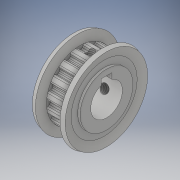
# Autodesk Inventor part: MTP16XL025-A-N12_b
Saved by Autodesk Inventor 2019 (Build 230136000, 136)
## iProperties
Created: 2023-12-31
Part Number: MTP16XL025-A-N12_b
Material: Generic
Catalog Web Link: www.cadenas.de
Description: ATP__XL025, ATP__XL031, ATP__ XL037, ATP__XL050, BTP__XL025, BTP__XL031, BTP__XL037, BTP__XL050, KTP__XL025, KTP__XL031, KTP__ XL037, KTP__XL050, NTP__XL025, NTP__XL031, NTP__ XL037, NTP__XL050, MTP__XL025, MTP__ XL037, MTP__XL050, MTPB__XL025, MTPB__ XL037, MTPB__XL050, MTPP__XL025, MTPP__ XL037, MTPP__XL050, STP__XL025, STP__XL031, STP__ XL037, STP__XL050, KATP__XL025, KATP__XL031, KATP__ XL037, KATP__XL050, KKTP__XL025, KKTP__XL031, KKTP__ XL037, KKTP__XL050_body-Timing Pulleys XL Type
Vendor: MISUMI
Document SubType Name: Modeling
Designer: psAdmin
Manufacturer: MISUMI
Mass: 4.98288 g
Surface Area: 37.8278 cm^2
Volume: 4.98288 cm^3
Density: 1 g/cm^3
Appearance: PSOLRGB-175-175-175
Category: PARTsolutions
Company: MISUMI
Title: MTP16XL025-A-N12
Author: Cadenas PARTsolutions
Comments: Timing Pulleys XL Type
PSOL_IDENT_0: {$CADENAS_DATA/23d-libs/misumi/metric/51_timing_pulleys/mtp_xl/mtp_xl.prj},887 {VTYP=3D},{NB=MTP16XL
PSOL_IDENT_1: 025-A-N12_b},{LINA=MTP16XL025-A-N12},{NN=ATP__XL025, ATP__XL031, ATP__ XL037, ATP__XL050, BTP__XL025
PSOL_IDENT_2: , BTP__XL031, BTP__XL037, BTP__XL050, KTP__XL025, KTP__XL031, KTP__ XL037, KTP__XL050, NTP__XL025, N
PSOL_IDENT_3: TP__XL031, NTP__ XL037, NTP__XL050, MTP__XL025, MTP__ XL037, MTP__XL050, MTPB__XL025, MTPB__ XL037,
PSOL_IDENT_4: MTPB__XL050, MTPP__XL025, MTPP__ XL037, MTPP__XL050, STP__XL025, STP__XL031, STP__ XL037, STP__XL050
PSOL_IDENT_5: , KATP__XL025, KATP__XL031, KATP__ XL037, KATP__XL050, KKTP__XL025, KKTP__XL031, KKTP__ XL037, KKTP_
PSOL_IDENT_6: _XL050_body},{DATE=06.01.2023 09:07:12},{GEOMDATE=06.01.2023 09:06:51},{VERSION=},{LINEID=30},{WBVAR=
PSOL_IDENT_7: MATP,ST,TNW,PS,SBS,DD,Z,J,Q,R,S,T,ALT1,ALT2,M,QSC,QFC,QTC,ALT3,K,KSC,KFC,KTC,ALT4,ZM,ZSC,ZFC,ZTC,ALT
PSOL_IDENT_8: 5,ALT6,ALT7,FC,ALT8,SRG,ALT9,BTC,TL,ALT10,TPC,ALT11,BC,ALT12,SLH,ALT13,BN},{WBNUMERIC=DD,Z,J,Q,R,S,T
PSOL_IDENT_9: ,QSC,QFC,QTC,K,KSC,KFC,KTC,ZSC,ZFC,ZTC,FC,SRG,BTC,TL,BC,SLH,BN}  {NB=MTP16XL025-A-N12_b},{LINA=MTP16
PSOL_IDENT_10: XL025-A-N12},{KT=DUMMY},{PN=MTP16XL025-A-N12},{TYPE=MTP},{MATP=S45C},{MATPALG= 'A2017','Aluminum All
PSOL_IDENT_11: oy 2000 series','S45C','1045 Carbon Steel Equivalent','SUS304','SUS304', 'A6000', '6000 Series Alumi
PSOL_IDENT_12: num Alloy' },{ST=-},{STALG= '-','-','BO','Black Oxide','ENP','Electroless Nickel Plating' },{NT=16},
PSOL_IDENT_13: {TNW=XL025},{TNWALG= 'XL025','XL031','XL037','XL050' },{BW=6.4mm (1/4inch)},{PS=A},{PSALG= 'A','B' }
PSOL_IDENT_14: ,{SBS=N},{SBSALG= 'H','Round Hole','P','Round Hole + Tap','N','New JIS Keywayed Bore + Tap (Standard
PSOL_IDENT_15: )','NK','New JIS Keywayed Bore + Tap (width 4.0mm, height 1.8mm)','C','Old JIS Keywayed Bore + Tap','
PSOL_IDENT_16: V','Stepped Hole','Y','Both Ends Stepped Hole','WB','Double Stepped Hole' },{DD=12.00},{DDALG=[8:8/1
PSOL_IDENT_17: ],[10:13/1]},{DDHA=[5:6/1],6.35,[7:12/1],12.7,[13:16/1]},{DDPA=[5:6/1],6.35,[7:12/1],12.7,[13:13/1]}
PSOL_IDENT_18: ,{DDNA=[8:8/1],[10:13/1]},{DDNK=[10:10/1]},{DDCA=[10,12]},{DDVA=[5:6/1],6.35,[7:12/1],12.7,[13:14/1]
PSOL_IDENT_19: },{DDY=[5:14/1]},{DDWB=[5:12/1]},{DDHB=},{DDPB=},{DDNB=},{DDCB=},{DDVFB=},{Z=0},{ZALG=[0]},{ZMIN=14.
PSOL_IDENT_20: 000},{ZAMAX=16.000},{ZBMAX=0.000},{DDZ=12.000},{J=0.0},{JALG=[0]},{JMIN=2.000},{JMAX=10.5},{JPN=},{Q=
PSOL_IDENT_21: 0},{QALG=[0]},{QRMIN=14.000},{QRMAX=16},{WBQMIN=16.000},{R=0},{RALG=[0]},{WBRMAX=-2.000},{S=0.0},{SA
PSOL_IDENT_22: LG=[0]},{SMAX=6.5},{T=0.0},{TALG=[0]},{TMAX=8},{SBSPN=-N12},{A=7.5},{W=12.5},{L=0},{PD=25.87},{OD=25
PSOL_IDENT_23: .36},{D=0},{DALG=17.000},{DE=20},{F=32},{E=20},{TT=1.6},{BBK=4.000},{TTK=1.8},{ALT1=},{ANG=112.500},
PSOL_IDENT_24: {ALT1ALG= '','w/o KC90 (Set Screw Angle)','KC90','with KC90 (Set Screw Angle)' },{ALT1PN=},{ALT2=},{
PSOL_IDENT_25: ALT2ALG= '','Not applicable' },{M=N/A},{MALG= 'N/A' },{MFTALG= 'N/A' },{MSALG= 'N/A' },{M3D=0.000},{
PSOL_IDENT_26: KDML=0.000},{ML=0.000},{MUL=0.000},{PITCH=0.000},{QSC=0.0},{QSCALG=0},{QFC=0.0},{QFCALG=0},{QTC=0.0}
PSOL_IDENT_27: ,{QTCALG=0},{QPCDMIN=0.000},{QPCDMINALG=0.000},{QPCDMAX=16.000},{ALT2PN=},{TAP=0.000},{ALT3=},{ALT3A
PSOL_IDENT_28: LG= '','Not applicable' },{K=0.0},{KALG=0},{KMIN=4.000},{KFTMAX=0.000},{KSMAX=0.000},{KSC=0.0},{KSCA
PSOL_IDENT_29: LG=0},{KFC=0.0},{KFCALG=0},{KTC=0.0},{KTCALG=0},{KSCMIN=16.000},{KPCDMIN=16.000},{KPCDMAX=16.000},{A
PSOL_IDENT_30: LT3PN=},{ALT4=},{ALT4ALG= '','Not applicable' },{ALT4MIN=22.500},{ALT4MAX=9.500},{ZM=N/A},{ZMALG= 'N
PSOL_IDENT_31: /A' },{ZMFTALG= 'N/A' },{ZMSALG= 'N/A' },{ZMDD1=0.0},{ZMDD2=0.0},{ZMHH=0.0},{ZSC=0.0},{ZSCALG=[0]},{
PSOL_IDENT_32: ZFC=0.0},{ZFCALG=[0]},{ZTC=0.0},{ZTCALG=[0]},{ZPCDMIN=0.000},{ZPCDMINALG=0.000},{ZPCDMAX=16.000},{AL
PSOL_IDENT_33: T4PN=},{ALT5=},{ALT5ALG= '','w/o Flange not Attached','NFC','with NFC (Flange not Attached)' },{ALT5
PSOL_IDENT_34: PN=},{ALT6=},{ALT6ALG= '','w/o Flange Attached on One Side Only','RFC','with RFC (Flange Attached on
PSOL_IDENT_35: The Boss Side Only)','LFC','with LFC (Flange Attached on The Opposite Side Only)' },{ALT6PN=},{ALT7=
PSOL_IDENT_36: },{ALT7ALG= '','w/o FC (Flange Cut)','FC','with FC (Flange Cut)' },{FC=0.0},{FCALG=0},{FCMIN=26.5},{
PSOL_IDENT_37: FCMAX=30.0},{ALT7PN=},{ALT8=},{ALT8ALG= '','Not applicable' },{ALT8ALGALG=16.000},{ALT8DD2=0.000},{A
PSOL_IDENT_38: LT8MM=0.000},{ALT8NN=0.000},{QC=0.000},{KC=0.000},{ZC=0.000},{SRG=0.0},{SRGALG=[0]},{SRGMAX=0.000},{
PSOL_IDENT_39: DD2=0.0},{MM=0.00},{NN=0.00},{ALT8PN=},{ALT9=},{ALT9ALG= '','Not applicable' },{BTC9=14.000},{TL9=1.
PSOL_IDENT_40: 000},{BTC=0},{BTCALG=[0]},{TL=0.0},{TLALG=0},{TLMIN=1.000},{TLMAX=-13.000},{BTCL=0},{BTCD=0},{ALT9PN=
PSOL_IDENT_41: },{WLBCTL=12.500},{ALT10=},{ALT10ALG= '','w/o TPC (Tapped Hole Dimension)','TPC','with TPC (Tapped H
PSOL_IDENT_42: ole Dimension)' },{TPC=N/A},{TPCALG= 'N/A' },{TPCM=4.000},{ALT10PN=},{ALT11=},{ALT11ALG= '','Not app
PSOL_IDENT_43: licable' },{BC=0.0},{BCALG=0},{BCMIN=7},{BCMAX=-13},{M1WBC=6.25},{ALT11PN=},{KTT=4.88},{ALT12=},{ALT
PSOL_IDENT_44: 12ALG= '','w/o SLH (Set Screw Length)','SLH','with SLH (Set Screw Length)' },{SLHALG=[0]},{SLH=0},{A
PSOL_IDENT_45: LT12PN=},{ALT13=},{ALT13ALG= '', 'Not applicable' },{BN=0.0},{BNALG=0},{BNMIN=-12},{BNMAX=-2.5},{ALT
PSOL_IDENT_46: 13PN=},{AC=M4x3},{M1=4.000},{M1L=3.000},{KEYA=1.000},{KEYB=0.000},{KEYM=1.000}
NB: MTP16XL025-A-N12_b
NN: 0
NT: 16
NBSYN: $PN._b
LINA: MTP16XL025-A-N12
CATALOG: Misumi
PN: MTP16XL025-A-N12
MATP: 1045 Carbon Steel Equivalent
ST: -
TNW: XL025
BW: 6.4mm (1/4inch)
PS: A
SBS: New JIS Keywayed Bore + Tap (Standard)
DD: 12
Z: 0
J: 0
Q: 0
R: 0
S: 0
T: 0
A: 7.5
W: 12.5
L: 0
PD: 25.87
OD: 25.36
D: 0
F: 32
E: 20
TT: 1.6
ALT1: w/o KC90 (Set Screw Angle)
ALT2: Not applicable
M: N/A
QSC: 0
QFC: 0
QTC: 0
ALT3: Not applicable
K: 0
KSC: 0
KFC: 0
KTC: 0
ALT4: Not applicable
ZM: N/A
ZMDD1: 0
ZMDD2: 0
ZMHH: 0
ZSC: 0
ZFC: 0
ZTC: 0
ALT5: w/o Flange not Attached
ALT6: w/o Flange Attached on One Side Only
ALT7: w/o FC (Flange Cut)
FC: 0
ALT8: Not applicable
SRG: 0
DD2: 0
MM: 0
ALT9: Not applicable
BTC: 0
TL: 0
BTCL: 0
BTCD: 0
ALT10: w/o TPC (Tapped Hole Dimension)
TPC: N/A
ALT11: Not applicable
BC: 0
ALT12: w/o SLH (Set Screw Length)
SLH: 0
ALT13: Not applicable
BN: 0
AC: M4x3
SUPPLIER: MISUMI
ARTICLENO: MTP16XL025-A-N12_b
BOMINFO: MTP16XL025-A-N12
CREATOR: CADENAS GmbH
Autodesk Inventor part; units mm, degrees
sketch "_____2" plane through (0, 0, 0) normal (0, 0, 1) x (1, 0, 0)
  line L0 (12.5, 0) -> (0, 0)
  line L1 (0, 0) -> (0, 10)
  line L2 (0, 10) -> (0.9, 10)
  line L3 (0.9, 10) -> (0.9, 12.469356)
  line L4 (0.9, 12.469356) -> (0.064927, 15.58589)
  line L5 (0.064927, 15.58589) -> (1.610409, 16)
  line L6 (1.610409, 16) -> (2.5, 12.68)
  line L7 (2.5, 12.68) -> (10, 12.68)
  line L8 (10, 12.68) -> (10.889591, 16)
  line L9 (10.889591, 16) -> (12.435073, 15.58589)
  line L10 (12.435073, 15.58589) -> (11.6, 12.469356)
  line L11 (11.6, 12.469356) -> (11.6, 10)
  line L12 (11.6, 10) -> (12.5, 10)
  line L13 (12.5, 10) -> (12.5, 0)
  line L14 (12.5, 0) -> (0, 0)
  constraints: 30 end point
revolve "Revolution1" add sketch "_____2" angle 360 about axis through (12.5, 0, 0) along (1, 0, 0)
sketch "Sketch2" plane through (12.5, 0, 0) normal (1, 0, 0) x (0, 0, -1)
  point P0 (0, 0)
hole "Hole1" at (12.5, 0, 0) direction (-1, 0, 0) diameter 12 depth 12.5
sketch "_____6" plane through (2.5, 0, 0) normal (1, 0, 0) x (0, 0, -1)
  arc A0 (-12.686458, 2.523493) -> (-12.686458, -2.523493) centre (0, 0) ccw
  arc A1 (-12.686458, -2.523493) -> (-10.755059, -7.186301) centre (0, 0) ccw
  arc A2 (-10.755059, -7.186301) -> (-7.186301, -10.755059) centre (0, 0) ccw
  arc A3 (-7.186301, -10.755059) -> (-2.523493, -12.686458) centre (0, 0) ccw
  arc A4 (-2.523493, -12.686458) -> (2.523493, -12.686458) centre (0, 0) ccw
  arc A5 (2.523493, -12.686458) -> (7.186301, -10.755059) centre (0, 0) ccw
  arc A6 (7.186301, -10.755059) -> (10.755059, -7.186301) centre (0, 0) ccw
  arc A7 (10.755059, -7.186301) -> (12.686458, -2.523493) centre (0, 0) ccw
  arc A8 (12.686458, -2.523493) -> (12.686458, 2.523493) centre (0, 0) ccw
  arc A9 (12.686458, 2.523493) -> (10.755059, 7.186301) centre (0, 0) ccw
  arc A10 (10.755059, 7.186301) -> (7.186301, 10.755059) centre (0, 0) ccw
  arc A11 (7.186301, 10.755059) -> (2.523493, 12.686458) centre (0, 0) ccw
  arc A12 (2.523493, 12.686458) -> (-2.523493, 12.686458) centre (0, 0) ccw
  arc A13 (-2.523493, 12.686458) -> (-7.186301, 10.755059) centre (0, 0) ccw
  arc A14 (-7.186301, 10.755059) -> (-10.755059, 7.186301) centre (0, 0) ccw
  arc A15 (-10.755059, 7.186301) -> (-12.686458, 2.523493) centre (0, 0) ccw
  arc A16 (-12.216815, -1.080185) -> (-12.563409, -1.715564) centre (-11.959018, -1.633033) ccw
  arc A17 (-12.563409, -1.715564) -> (-12.436357, -2.473745) centre (0, 0) ccw
  arc A18 (-12.436357, -2.473745) -> (-12.263594, -3.222834) centre (0, 0) ccw
  arc A19 (-12.263594, -3.222834) -> (-11.700234, -3.677212) centre (-11.673626, -3.067792) ccw
  line L0 (-11.700234, -3.677212) -> (-11.052822, -3.705478)
  arc A20 (-10.511015, -4.093528) -> (-11.052822, -3.705478) centre (-11.079429, -4.314898) ccw
  arc A21 (-10.511015, -4.093528) -> (-10.326971, -4.537849) centre (0, 0) ccw
  arc A22 (-10.435694, -5.195356) -> (-10.326971, -4.537849) centre (-10.885433, -4.783246) ccw
  line L1 (-10.435694, -5.195356) -> (-10.873496, -5.673133)
  arc A23 (-10.873496, -5.673133) -> (-10.950558, -6.392783) centre (-10.423757, -6.085244) ccw
  arc A24 (-10.950558, -6.392783) -> (-10.543035, -7.044631) centre (0, 0) ccw
  arc A25 (-10.543035, -7.044631) -> (-10.096758, -7.670585) centre (0, 0) ccw
  arc A26 (-10.096758, -7.670585) -> (-9.402399, -7.874786) centre (-9.611031, -7.301574) ccw
  line L2 (-9.402399, -7.874786) -> (-8.79345, -7.653147)
  arc A27 (-8.144386, -7.804318) -> (-8.79345, -7.653147) centre (-8.584818, -8.22636) ccw
  arc A28 (-8.144386, -7.804318) -> (-7.804318, -8.144386) centre (0, 0) ccw
  arc A29 (-7.653147, -8.79345) -> (-7.804318, -8.144386) centre (-8.22636, -8.584818) ccw
  line L3 (-7.653147, -8.79345) -> (-7.874786, -9.402399)
  arc A30 (-7.874786, -9.402399) -> (-7.670585, -10.096758) centre (-7.301574, -9.611031) ccw
  arc A31 (-7.670585, -10.096758) -> (-7.044631, -10.543035) centre (0, 0) ccw
  arc A32 (-7.044631, -10.543035) -> (-6.392783, -10.950558) centre (0, 0) ccw
  arc A33 (-6.392783, -10.950558) -> (-5.673133, -10.873496) centre (-6.085244, -10.423757) ccw
  line L4 (-5.673133, -10.873496) -> (-5.195356, -10.435694)
  arc A34 (-4.537848, -10.326971) -> (-5.195356, -10.435694) centre (-4.783246, -10.885433) ccw
  arc A35 (-4.537848, -10.326971) -> (-4.093528, -10.511015) centre (0, 0) ccw
  arc A36 (-3.705478, -11.052822) -> (-4.093528, -10.511015) centre (-4.314898, -11.079429) ccw
  line L5 (-3.705478, -11.052822) -> (-3.677212, -11.700234)
  arc A37 (-3.677212, -11.700234) -> (-3.222834, -12.263594) centre (-3.067792, -11.673626) ccw
  arc A38 (-3.222834, -12.263594) -> (-2.473745, -12.436357) centre (0, 0) ccw
  arc A39 (-2.473745, -12.436357) -> (-1.715564, -12.563409) centre (0, 0) ccw
  arc A40 (-1.715564, -12.563409) -> (-1.080185, -12.216815) centre (-1.633033, -11.959018) ccw
  line L6 (-1.080185, -12.216815) -> (-0.806316, -11.629501)
  arc A41 (-0.240464, -11.277437) -> (-0.806316, -11.629501) centre (-0.253468, -11.887298) ccw
  arc A42 (-0.240464, -11.277437) -> (0.240464, -11.277437) centre (0, 0) ccw
  arc A43 (0.806316, -11.629501) -> (0.240464, -11.277437) centre (0.253468, -11.887298) ccw
  line L7 (0.806316, -11.629501) -> (1.080185, -12.216815)
  arc A44 (1.080185, -12.216815) -> (1.715564, -12.563409) centre (1.633033, -11.959018) ccw
  arc A45 (1.715564, -12.563409) -> (2.473745, -12.436357) centre (0, 0) ccw
  arc A46 (2.473745, -12.436357) -> (3.222834, -12.263594) centre (0, 0) ccw
  arc A47 (3.222834, -12.263594) -> (3.677212, -11.700234) centre (3.067792, -11.673626) ccw
  line L8 (3.677212, -11.700234) -> (3.705478, -11.052822)
  arc A48 (4.093528, -10.511015) -> (3.705478, -11.052822) centre (4.314898, -11.079429) ccw
  arc A49 (4.093528, -10.511015) -> (4.537849, -10.326971) centre (0, 0) ccw
  arc A50 (5.195356, -10.435694) -> (4.537849, -10.326971) centre (4.783246, -10.885433) ccw
  line L9 (5.195356, -10.435694) -> (5.673133, -10.873496)
  arc A51 (5.673133, -10.873496) -> (6.392783, -10.950558) centre (6.085244, -10.423757) ccw
  arc A52 (6.392783, -10.950558) -> (7.044631, -10.543035) centre (0, 0) ccw
  arc A53 (7.044631, -10.543035) -> (7.670585, -10.096758) centre (0, 0) ccw
  arc A54 (7.670585, -10.096758) -> (7.874786, -9.402399) centre (7.301574, -9.611031) ccw
  line L10 (7.874786, -9.402399) -> (7.653147, -8.79345)
  arc A55 (7.804318, -8.144386) -> (7.653147, -8.79345) centre (8.22636, -8.584818) ccw
  arc A56 (7.804318, -8.144386) -> (8.144386, -7.804318) centre (0, 0) ccw
  arc A57 (8.79345, -7.653147) -> (8.144386, -7.804318) centre (8.584818, -8.22636) ccw
  line L11 (8.79345, -7.653147) -> (9.402399, -7.874786)
  arc A58 (9.402399, -7.874786) -> (10.096758, -7.670585) centre (9.611031, -7.301574) ccw
  arc A59 (10.096758, -7.670585) -> (10.543035, -7.044631) centre (0, 0) ccw
  arc A60 (10.543035, -7.044631) -> (10.950558, -6.392783) centre (0, 0) ccw
  arc A61 (10.950558, -6.392783) -> (10.873496, -5.673133) centre (10.423757, -6.085244) ccw
  line L12 (10.873496, -5.673133) -> (10.435694, -5.195356)
  arc A62 (10.326971, -4.537848) -> (10.435694, -5.195356) centre (10.885433, -4.783246) ccw
  arc A63 (10.326971, -4.537848) -> (10.511015, -4.093528) centre (0, 0) ccw
  arc A64 (11.052822, -3.705478) -> (10.511015, -4.093528) centre (11.079429, -4.314898) ccw
  line L13 (11.052822, -3.705478) -> (11.700234, -3.677212)
  arc A65 (11.700234, -3.677212) -> (12.263594, -3.222834) centre (11.673626, -3.067792) ccw
  arc A66 (12.263594, -3.222834) -> (12.436357, -2.473745) centre (0, 0) ccw
  arc A67 (12.436357, -2.473745) -> (12.563409, -1.715564) centre (0, 0) ccw
  arc A68 (12.563409, -1.715564) -> (12.216815, -1.080185) centre (11.959018, -1.633033) ccw
  line L14 (12.216815, -1.080185) -> (11.629501, -0.806316)
  arc A69 (11.277437, -0.240464) -> (11.629501, -0.806316) centre (11.887298, -0.253468) ccw
  arc A70 (11.277437, -0.240464) -> (11.277437, 0.240464) centre (0, 0) ccw
  arc A71 (11.629501, 0.806316) -> (11.277437, 0.240464) centre (11.887298, 0.253468) ccw
  line L15 (11.629501, 0.806316) -> (12.216815, 1.080185)
  arc A72 (12.216815, 1.080185) -> (12.563409, 1.715564) centre (11.959018, 1.633033) ccw
  arc A73 (12.563409, 1.715564) -> (12.436357, 2.473745) centre (0, 0) ccw
  arc A74 (12.436357, 2.473745) -> (12.263594, 3.222834) centre (0, 0) ccw
  arc A75 (12.263594, 3.222834) -> (11.700234, 3.677212) centre (11.673626, 3.067792) ccw
  line L16 (11.700234, 3.677212) -> (11.052822, 3.705478)
  arc A76 (10.511015, 4.093528) -> (11.052822, 3.705478) centre (11.079429, 4.314898) ccw
  arc A77 (10.511015, 4.093528) -> (10.326971, 4.537848) centre (0, 0) ccw
  arc A78 (10.435694, 5.195356) -> (10.326971, 4.537848) centre (10.885433, 4.783246) ccw
  line L17 (10.435694, 5.195356) -> (10.873496, 5.673133)
  arc A79 (10.873496, 5.673133) -> (10.950558, 6.392783) centre (10.423757, 6.085244) ccw
  arc A80 (10.950558, 6.392783) -> (10.543035, 7.044631) centre (0, 0) ccw
  arc A81 (10.543035, 7.044631) -> (10.096758, 7.670585) centre (0, 0) ccw
  arc A82 (10.096758, 7.670585) -> (9.402399, 7.874786) centre (9.611031, 7.301574) ccw
  line L18 (9.402399, 7.874786) -> (8.79345, 7.653147)
  arc A83 (8.144386, 7.804318) -> (8.79345, 7.653147) centre (8.584818, 8.22636) ccw
  arc A84 (8.144386, 7.804318) -> (7.804318, 8.144386) centre (0, 0) ccw
  arc A85 (7.653147, 8.79345) -> (7.804318, 8.144386) centre (8.22636, 8.584818) ccw
  line L19 (7.653147, 8.79345) -> (7.874786, 9.402399)
  arc A86 (7.874786, 9.402399) -> (7.670585, 10.096758) centre (7.301574, 9.611031) ccw
  arc A87 (7.670585, 10.096758) -> (7.044631, 10.543035) centre (0, 0) ccw
  arc A88 (7.044631, 10.543035) -> (6.392783, 10.950558) centre (0, 0) ccw
  arc A89 (6.392783, 10.950558) -> (5.673133, 10.873496) centre (6.085244, 10.423757) ccw
  line L20 (5.673133, 10.873496) -> (5.195356, 10.435694)
  arc A90 (4.537848, 10.326971) -> (5.195356, 10.435694) centre (4.783246, 10.885433) ccw
  arc A91 (4.537848, 10.326971) -> (4.093528, 10.511015) centre (0, 0) ccw
  arc A92 (3.705478, 11.052822) -> (4.093528, 10.511015) centre (4.314898, 11.079429) ccw
  line L21 (3.705478, 11.052822) -> (3.677212, 11.700234)
  arc A93 (3.677212, 11.700234) -> (3.222834, 12.263594) centre (3.067792, 11.673626) ccw
  arc A94 (3.222834, 12.263594) -> (2.473745, 12.436357) centre (0, 0) ccw
  arc A95 (2.473745, 12.436357) -> (1.715564, 12.563409) centre (0, 0) ccw
  arc A96 (1.715564, 12.563409) -> (1.080185, 12.216815) centre (1.633033, 11.959018) ccw
  line L22 (1.080185, 12.216815) -> (0.806316, 11.629501)
  arc A97 (0.240465, 11.277437) -> (0.806316, 11.629501) centre (0.253468, 11.887298) ccw
  arc A98 (0.240465, 11.277437) -> (-0.240465, 11.277437) centre (0, 0) ccw
  arc A99 (-0.806316, 11.629501) -> (-0.240465, 11.277437) centre (-0.253468, 11.887298) ccw
  line L23 (-0.806316, 11.629501) -> (-1.080185, 12.216815)
  arc A100 (-1.080185, 12.216815) -> (-1.715564, 12.563409) centre (-1.633033, 11.959018) ccw
  arc A101 (-1.715564, 12.563409) -> (-2.473745, 12.436357) centre (0, 0) ccw
  arc A102 (-2.473745, 12.436357) -> (-3.222834, 12.263594) centre (0, 0) ccw
  arc A103 (-3.222834, 12.263594) -> (-3.677212, 11.700234) centre (-3.067792, 11.673626) ccw
  line L24 (-3.677212, 11.700234) -> (-3.705478, 11.052822)
  arc A104 (-4.093528, 10.511015) -> (-3.705478, 11.052822) centre (-4.314898, 11.079429) ccw
  arc A105 (-4.093528, 10.511015) -> (-4.537849, 10.326971) centre (0, 0) ccw
  arc A106 (-5.195356, 10.435694) -> (-4.537849, 10.326971) centre (-4.783246, 10.885433) ccw
  line L25 (-5.195356, 10.435694) -> (-5.673133, 10.873496)
  arc A107 (-5.673133, 10.873496) -> (-6.392783, 10.950558) centre (-6.085244, 10.423757) ccw
  arc A108 (-6.392783, 10.950558) -> (-7.044631, 10.543035) centre (0, 0) ccw
  arc A109 (-7.044631, 10.543035) -> (-7.670585, 10.096758) centre (0, 0) ccw
  arc A110 (-7.670585, 10.096758) -> (-7.874786, 9.402399) centre (-7.301574, 9.611031) ccw
  line L26 (-7.874786, 9.402399) -> (-7.653147, 8.79345)
  arc A111 (-7.804318, 8.144386) -> (-7.653147, 8.79345) centre (-8.22636, 8.584818) ccw
  arc A112 (-7.804318, 8.144386) -> (-8.144386, 7.804318) centre (0, 0) ccw
  arc A113 (-8.79345, 7.653147) -> (-8.144386, 7.804318) centre (-8.584818, 8.22636) ccw
  line L27 (-8.79345, 7.653147) -> (-9.402399, 7.874786)
  arc A114 (-9.402399, 7.874786) -> (-10.096758, 7.670585) centre (-9.611031, 7.301574) ccw
  arc A115 (-10.096758, 7.670585) -> (-10.543035, 7.044631) centre (0, 0) ccw
  arc A116 (-10.543035, 7.044631) -> (-10.950558, 6.392783) centre (0, 0) ccw
  arc A117 (-10.950558, 6.392783) -> (-10.873496, 5.673133) centre (-10.423757, 6.085244) ccw
  line L28 (-10.873496, 5.673133) -> (-10.435694, 5.195356)
  arc A118 (-10.326971, 4.537848) -> (-10.435694, 5.195356) centre (-10.885433, 4.783246) ccw
  arc A119 (-10.326971, 4.537848) -> (-10.511015, 4.093528) centre (0, 0) ccw
  arc A120 (-11.052822, 3.705478) -> (-10.511015, 4.093528) centre (-11.079429, 4.314898) ccw
  line L29 (-11.052822, 3.705478) -> (-11.700234, 3.677212)
  arc A121 (-11.700234, 3.677212) -> (-12.263594, 3.222834) centre (-11.673626, 3.067792) ccw
  arc A122 (-12.263594, 3.222834) -> (-12.436357, 2.473745) centre (0, 0) ccw
  arc A123 (-12.436357, 2.473745) -> (-12.563409, 1.715564) centre (0, 0) ccw
  arc A124 (-12.563409, 1.715564) -> (-12.216815, 1.080185) centre (-11.959018, 1.633033) ccw
  line L30 (-12.216815, 1.080185) -> (-11.629501, 0.806316)
  arc A125 (-11.277437, 0.240465) -> (-11.629501, 0.806316) centre (-11.887298, 0.253468) ccw
  arc A126 (-11.277437, 0.240465) -> (-11.277437, -0.240465) centre (0, 0) ccw
  arc A127 (-11.629501, -0.806316) -> (-11.277437, -0.240465) centre (-11.887298, -0.253468) ccw
  line L31 (-11.629501, -0.806316) -> (-12.216815, -1.080185)
  constraints: 256 point on circle, 128 centre point, 64 end point
extrude "Extrusion1" cut sketch "_____6" along normal blind 7.5
sketch "_____43" plane through (0, 0, 0) normal (1, 0, 0) x (0, 0, -1)
  line L0 (-2, 7.8) -> (-2, 0)
  line L1 (-2, 0) -> (2, 0)
  line L2 (2, 0) -> (2, 7.8)
  line L3 (2, 7.8) -> (-2, 7.8)
  constraints: 8 end point
extrude "Extrusion2" cut sketch "_____43" along normal blind 12.5
sketch "_____15" plane through (6.25, 0, 0) normal (1, 0, 0) x (0, 0, -1)
  line L0 (0, 0) -> (0, 12.68)
  line L1 (0, 12.68) -> (1.621, 12.68)
  line L2 (1.621, 12.68) -> (1.621, 0)
  line L3 (1.621, 0) -> (0, 0)
  line L4 (0, 0) -> (0, 12.68)
  constraints: 10 end point
revolve "Revolution2" cut sketch "_____15" angle 360 about axis through (6.25, 0, 0) along (0, -1, 0)
thread "Thread1" size "M4x0.7" class "6H" standard "ISO Metric profile" length 4.88
sketch "_____16" plane through (6.25, 0, 0) normal (1, 0, 0) x (0, 0, -1)
  line L0 (0, 0) -> (11.714792, -4.852426)
  line L1 (11.714792, -4.852426) -> (11.094463, -6.350035)
  line L2 (11.094463, -6.350035) -> (-0.62033, -1.497609)
  line L3 (-0.62033, -1.497609) -> (0, 0)
  line L4 (0, 0) -> (11.714792, -4.852426)
  constraints: 10 end point
revolve "Revolution3" cut sketch "_____16" angle 360 about axis through (6.25, 0, 0) along (0, 0.3826834, 0.9238795)
thread "Thread2" size "M4x0.7" class "6H" standard "ISO Metric profile" length 6.68
ref_plane "to_screw1_XY" through (6.25, 7.8, 0) normal (0, 1, 0) x (1, 0, 0)
ref_plane "to_screw1_YZ" through (6.25, 7.8, 0) normal (1, 0, 0) x (0, 0, -1)
ref_plane "to_screw1_ZX" through (6.25, 7.8, 0) normal (0, 0, -1) x (0, 1, 0)
ref_plane "to_screw2_XY" through (6.25, -2.296101, -5.543277) normal (0, -0.3826834, -0.9238795) x (1, 0, 0)
ref_plane "to_screw2_YZ" through (6.25, -2.296101, -5.543277) normal (1, 0, 0) x (0, -0.9238795, 0.3826834)
ref_plane "to_screw2_ZX" through (6.25, -2.296101, -5.543277) normal (0, -0.9238795, 0.3826834) x (0, -0.3826834, -0.9238795)
body "Solid1"
